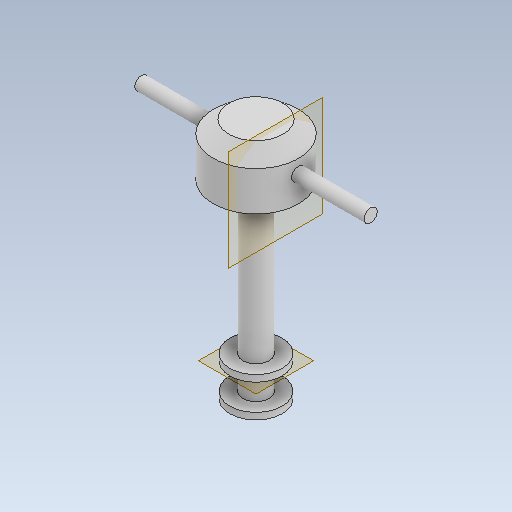
# Autodesk Inventor part: capistan upper
Saved by Autodesk Inventor 2020.2 (Build 242310000, 310)
## iProperties
Created: 2021-01-28
Part Number: capistan upper
Material: Generic
Document SubType Name: Modeling
Designer: con_c_000
Density: 1 g/cm^3
Appearance: Default
Author: con_c_000
Autodesk Inventor part; units mm, degrees
ref_plane "YZ Plane" through (0, 0, 0) normal (1, 0, 0) x (0, 1, 0)
ref_plane "XZ Plane" through (0, 0, 0) normal (0, 1, 0) x (-1, 0, 0)
ref_plane "XY Plane" through (0, 0, 0) normal (0, 0, 1) x (1, 0, 0)
sketch "Sketch1" plane through (0, 0, 0) normal (0, 1, 0) x (-1, 0, 0)
  circle A0 centre (0, 0) radius 152.4
  circle A1 centre (0, 0) radius 165.1
  dimension "d0" = 304.8
  dimension "d1" = 330.2
  constraints: 2 centre point, 2 coincident
  measures "d0" diameter of A0
  measures "d1" diameter of A1
extrude "Extrusion1" add sketch "Sketch1" along normal blind 152.4
sketch "Sketch2" plane through (0, 0, 0) normal (1, 0, 0) x (0, 1, 0)
  circle A0 centre (100.6077, 0) radius 25.4
  point P0 (0, 0)
  dimension "d4" = 50.8
  constraints: 1 centre point
  measures "d4" diameter of A0
extrude "Extrusion2" add sketch "Sketch2" along normal mid plane 889
sketch "Sketch4" plane through (0, 152.4, 0) normal (0, 1, 0) x (1, 0, 0)
  circle A0 centre (0, 0) radius 152.4
  constraints: 1 centre point, 1 coincident
extrude "Extrusion4" cut sketch "Sketch4" against normal through all
sketch "Sketch5" plane through (0, 152.4, 0) normal (0, 1, 0) x (1, 0, 0)
  circle A0 centre (0, 0) radius 165.1
  constraints: 1 centre point, 1 coincident
extrude "Extrusion5" add sketch "Sketch5" along normal blind 50.8 draft -50
sketch "Sketch6" plane through (0, 152.4, 0) normal (0, -1, 0) x (1, 0, 0)
  circle A0 centre (0, 0) radius 104.5589 projected
  circle A1 centre (0, 0) radius 50.8
  dimension "d15" = 101.6
  constraints: 1 centre point, 1 coincident
  measures "d15" diameter of A1
extrude "Extrusion6" add sketch "Sketch6" along normal blind 863.6 contours A1
sketch "Sketch7" plane through (0, -711.2, 0) normal (0, -1, 0) x (1, 0, 0)
  circle A0 centre (0, 0) radius 104.5589 projected
  circle A1 centre (0, 0) radius 101.6
  dimension "d18" = 203.2
  constraints: 1 centre point, 1 coincident
  measures "d18" diameter of A1
extrude "Extrusion7" add sketch "Sketch7" along normal blind 25.4 contours A1
ref_plane "Work Plane1" through (0, -609.6, 0) normal (0, 1, 0) x (1, 0, 0)
sketch "Sketch8" plane through (0, -609.6, 0) normal (0, 1, 0) x (1, 0, 0)
  circle A0 centre (0, 0) radius 101.6
  dimension "d22" = 203.2
  constraints: 1 centre point, 1 coincident
  measures "d22" diameter of A0
extrude "Extrusion8" add sketch "Sketch8" along normal blind 25.4
ref_plane "Work Plane2" through (75.376, -18.8821, -44.9646) normal (1, 0, 0) x (0, 1, 0)
sketch "Sketch9" plane through (75.376, -18.8821, -44.9646) normal (1, 0, 0) x (0, 1, 0)
  circle A0 centre (-604.603, 44.9646) radius 12.7
  point P0 (18.8821, 44.9646)
  dimension "d25" = 25.4
  constraints: 1 centre point
  measures "d25" diameter of A0
extrude "Extrusion9" cut sketch "Sketch9" against normal through all
body "Solid1"
